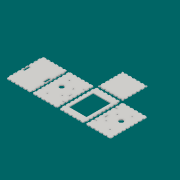
# Autodesk Inventor part: panelsWithKerf
Saved by Autodesk Inventor 2016 (Build 200138000, 138)
## iProperties
Created: 2016-09-07
Part Number: panelsWithKerf
Material: Generic
Document SubType Name: Modeling
Designer: sawaiz
Density: 1 g/cm^3
Appearance: Default
Author: sawaiz
Autodesk Inventor part; units mm, degrees
(part 1 of 2)
ref_plane "YZ Plane" through (0, 0, 0) normal (1, 0, 0) x (0, 1, 0)
ref_plane "XZ Plane" through (0, 0, 0) normal (0, 1, 0) x (-1, 0, 0)
ref_plane "XY Plane" through (0, 0, 0) normal (0, 0, 1) x (1, 0, 0)
sketch "Sketch2" plane through (0, 0, 0) normal (0, 0, 1) x (1, 0, 0)
  line L0 (-304.6687, 15) -> (-304.6687, -15) construction
  line L1 (-304.6687, -15) -> (-314.6687, -15) construction
  line L2 (-314.6687, -15) -> (-314.6687, 15) construction
  line L3 (-314.6687, 15) -> (-304.6687, 15) construction
  line L4 (-204.6687, 15) -> (-204.6687, -15) construction
  line L5 (-204.6687, -15) -> (-214.6687, -15) construction
  line L6 (-214.6687, -15) -> (-214.6687, 15) construction
  line L7 (-214.6687, 15) -> (-204.6687, 15) construction
  circle A0 centre (-316.4937, -50) radius 1.7 projected
  circle A1 centre (-316.4937, 50) radius 1.7 projected
  circle A2 centre (-202.8437, -50) radius 1.7 projected
  circle A3 centre (-202.8437, 50) radius 1.7 projected
  line L8 (-316.4937, 86.825) -> (-316.4937, 75) construction
  line L9 (-316.4937, 75) -> (-319.6687, 75) construction
  line L10 (-319.6687, 75) -> (-319.6687, 65) construction
  line L11 (-319.6687, 65) -> (-316.4937, 65) construction
  line L12 (-316.4937, 65) -> (-316.4937, 55) construction
  line L13 (-316.4937, 55) -> (-319.6687, 55) construction
  line L14 (-319.6687, 55) -> (-319.6687, 45) construction
  line L15 (-319.6687, 45) -> (-316.4937, 45) construction
  line L16 (-316.4937, 45) -> (-316.4937, 35) construction
  line L17 (-316.4937, 35) -> (-319.6687, 35) construction
  line L18 (-319.6687, 35) -> (-319.6687, 25) construction
  line L19 (-319.6687, 25) -> (-316.4937, 25) construction
  line L20 (-316.4937, 25) -> (-316.4937, 15) construction
  line L21 (-316.4937, 15) -> (-319.6687, 15) construction
  line L22 (-319.6687, 15) -> (-319.6687, 5) construction
  line L23 (-319.6687, 5) -> (-316.4937, 5) construction
  line L24 (-316.4937, 5) -> (-316.4937, -5) construction
  line L25 (-316.4937, -5) -> (-319.6687, -5) construction
  line L26 (-319.6687, -5) -> (-319.6687, -15) construction
  line L27 (-319.6687, -15) -> (-316.4937, -15) construction
  line L28 (-316.4937, -15) -> (-316.4937, -25) construction
  line L29 (-316.4937, -25) -> (-319.6687, -25) construction
  line L30 (-319.6687, -25) -> (-319.6687, -35) construction
  line L31 (-319.6687, -35) -> (-316.4937, -35) construction
  line L32 (-316.4937, -35) -> (-316.4937, -45) construction
  line L33 (-316.4937, -45) -> (-319.6687, -45) construction
  line L34 (-319.6687, -45) -> (-319.6687, -55) construction
  line L35 (-319.6687, -55) -> (-316.4937, -55) construction
  line L36 (-316.4937, -55) -> (-316.4937, -65) construction
  line L37 (-316.4937, -65) -> (-319.6687, -65) construction
  line L38 (-319.6687, -65) -> (-319.6687, -75) construction
  line L39 (-319.6687, -75) -> (-316.4937, -75) construction
  line L40 (-316.4937, -75) -> (-316.4937, -86.825) construction
  line L41 (-316.4937, -86.825) -> (-314.6687, -86.825) construction
  line L42 (-314.6687, -86.825) -> (-314.6687, -90) construction
  line L43 (-314.6687, -90) -> (-304.6687, -90) construction
  line L44 (-304.6687, -90) -> (-304.6687, -86.825) construction
  line L45 (-304.6687, -86.825) -> (-294.6687, -86.825) construction
  line L46 (-294.6687, -86.825) -> (-294.6687, -90) construction
  line L47 (-294.6687, -90) -> (-284.6687, -90) construction
  line L48 (-284.6687, -90) -> (-284.6687, -86.825) construction
  line L49 (-284.6687, -86.825) -> (-274.6687, -86.825) construction
  line L50 (-274.6687, -86.825) -> (-274.6687, -90) construction
  line L51 (-274.6687, -90) -> (-264.6687, -90) construction
  line L52 (-264.6687, -90) -> (-264.6687, -86.825) construction
  line L53 (-264.6687, -86.825) -> (-254.6687, -86.825) construction
  line L54 (-254.6687, -86.825) -> (-254.6687, -90) construction
  line L55 (-254.6687, -90) -> (-244.6687, -90) construction
  line L56 (-244.6687, -90) -> (-244.6687, -86.825) construction
  line L57 (-244.6687, -86.825) -> (-234.6687, -86.825) construction
  line L58 (-234.6687, -86.825) -> (-234.6687, -90) construction
  line L59 (-234.6687, -90) -> (-224.6687, -90) construction
  line L60 (-224.6687, -90) -> (-224.6687, -86.825) construction
  line L61 (-224.6687, -86.825) -> (-214.6687, -86.825) construction
  line L62 (-214.6687, -86.825) -> (-214.6687, -90) construction
  line L63 (-214.6687, -90) -> (-204.6687, -90) construction
  line L64 (-204.6687, -90) -> (-204.6687, -86.825) construction
  line L65 (-204.6687, -86.825) -> (-202.8437, -86.825) construction
  line L66 (-202.8437, -86.825) -> (-202.8437, -75) construction
  line L67 (-202.8437, -75) -> (-199.6687, -75) construction
  line L68 (-199.6687, -75) -> (-199.6687, -65) construction
  line L69 (-199.6687, -65) -> (-202.8437, -65) construction
  line L70 (-202.8437, -65) -> (-202.8437, -55) construction
  line L71 (-202.8437, -55) -> (-199.6687, -55) construction
  line L72 (-199.6687, -55) -> (-199.6687, -45) construction
  line L73 (-199.6687, -45) -> (-202.8437, -45) construction
  line L74 (-202.8437, -45) -> (-202.8437, -35) construction
  line L75 (-202.8437, -35) -> (-199.6687, -35) construction
  line L76 (-199.6687, -35) -> (-199.6687, -25) construction
  line L77 (-199.6687, -25) -> (-202.8437, -25) construction
  line L78 (-202.8437, -25) -> (-202.8437, -15) construction
  line L79 (-202.8437, -15) -> (-199.6687, -15) construction
  line L80 (-199.6687, -15) -> (-199.6687, -5) construction
  line L81 (-199.6687, -5) -> (-202.8437, -5) construction
  line L82 (-202.8437, -5) -> (-202.8437, 5) construction
  line L83 (-202.8437, 5) -> (-199.6687, 5) construction
  line L84 (-199.6687, 5) -> (-199.6687, 15) construction
  line L85 (-199.6687, 15) -> (-202.8437, 15) construction
  line L86 (-202.8437, 15) -> (-202.8437, 25) construction
  line L87 (-202.8437, 25) -> (-199.6687, 25) construction
  line L88 (-199.6687, 25) -> (-199.6687, 35) construction
  line L89 (-199.6687, 35) -> (-202.8437, 35) construction
  line L90 (-202.8437, 35) -> (-202.8437, 45) construction
  line L91 (-202.8437, 45) -> (-199.6687, 45) construction
  line L92 (-199.6687, 45) -> (-199.6687, 55) construction
  line L93 (-199.6687, 55) -> (-202.8437, 55) construction
  line L94 (-202.8437, 55) -> (-202.8437, 65) construction
  line L95 (-202.8437, 65) -> (-199.6687, 65) construction
  line L96 (-199.6687, 65) -> (-199.6687, 75) construction
  line L97 (-199.6687, 75) -> (-202.8437, 75) construction
  line L98 (-202.8437, 75) -> (-202.8437, 86.825) construction
  line L99 (-202.8437, 86.825) -> (-204.6687, 86.825) construction
  line L100 (-204.6687, 86.825) -> (-204.6687, 90) construction
  line L101 (-204.6687, 90) -> (-214.6687, 90) construction
  line L102 (-214.6687, 90) -> (-214.6687, 86.825) construction
  line L103 (-214.6687, 86.825) -> (-224.6687, 86.825) construction
  line L104 (-224.6687, 86.825) -> (-224.6687, 90) construction
  line L105 (-224.6687, 90) -> (-234.6687, 90) construction
  line L106 (-234.6687, 90) -> (-234.6687, 86.825) construction
  line L107 (-234.6687, 86.825) -> (-244.6687, 86.825) construction
  line L108 (-244.6687, 86.825) -> (-244.6687, 90) construction
  line L109 (-244.6687, 90) -> (-254.6687, 90) construction
  line L110 (-254.6687, 90) -> (-254.6687, 86.825) construction
  line L111 (-254.6687, 86.825) -> (-264.6687, 86.825) construction
  line L112 (-264.6687, 86.825) -> (-264.6687, 90) construction
  line L113 (-264.6687, 90) -> (-274.6687, 90) construction
  line L114 (-274.6687, 90) -> (-274.6687, 86.825) construction
  line L115 (-274.6687, 86.825) -> (-284.6687, 86.825) construction
  line L116 (-284.6687, 86.825) -> (-284.6687, 90) construction
  line L117 (-284.6687, 90) -> (-294.6687, 90) construction
  line L118 (-294.6687, 90) -> (-294.6687, 86.825) construction
  line L119 (-294.6687, 86.825) -> (-304.6687, 86.825) construction
  line L120 (-304.6687, 86.825) -> (-304.6687, 90) construction
  line L121 (-304.6687, 90) -> (-314.6687, 90) construction
  line L122 (-314.6687, 90) -> (-314.6687, 86.825) construction
  line L123 (-314.6687, 86.825) -> (-316.4937, 86.825) construction
  line L124 (-87.1256, -13.335) -> (-90.9356, -13.335) projected
  line L125 (-90.9356, -13.335) -> (-90.9356, -1.905) projected
  line L126 (-90.9356, -1.905) -> (-87.1256, -1.905) projected
  line L127 (-87.1256, -1.905) -> (-87.1256, -13.335) projected
  circle A4 centre (-92.8406, -15.24) radius 1.078 projected
  circle A5 centre (-85.2206, 0) radius 1.078 projected
  circle A6 centre (-85.2206, -15.24) radius 1.078 projected
  circle A7 centre (-92.8406, 0) radius 1.078 projected
  line L128 (-76.1156, -48.5) -> (-74.1156, -48.5) construction
  line L129 (-74.1156, -48.5) -> (-74.1156, -45) construction
  line L130 (-74.1156, -45) -> (-70.9406, -45) construction
  line L131 (-70.9406, -45) -> (-70.9406, -35) construction
  line L132 (-70.9406, -35) -> (-74.1156, -35) construction
  line L133 (-74.1156, -35) -> (-74.1156, -25) construction
  line L134 (-74.1156, -25) -> (-70.9406, -25) construction
  line L135 (-70.9406, -25) -> (-70.9406, -15) construction
  line L136 (-70.9406, -15) -> (-74.1156, -15) construction
  line L137 (-74.1156, -15) -> (-74.1156, -5) construction
  line L138 (-74.1156, -5) -> (-70.9406, -5) construction
  line L139 (-70.9406, -5) -> (-70.9406, 5) construction
  line L140 (-70.9406, 5) -> (-74.1156, 5) construction
  line L141 (-74.1156, 5) -> (-74.1156, 15) construction
  line L142 (-74.1156, 15) -> (-70.9406, 15) construction
  line L143 (-70.9406, 15) -> (-70.9406, 25) construction
  line L144 (-70.9406, 25) -> (-74.1156, 25) construction
  line L145 (-74.1156, 25) -> (-74.1156, 35) construction
  line L146 (-74.1156, 35) -> (-70.9406, 35) construction
  line L147 (-70.9406, 35) -> (-70.9406, 45) construction
  line L148 (-70.9406, 45) -> (-74.1156, 45) construction
  line L149 (-74.1156, 45) -> (-74.1156, 48.5) construction
  line L150 (-74.1156, 48.5) -> (-76.1156, 48.5) construction
  line L151 (-76.1156, 48.5) -> (-76.1156, 47.25) construction
  line L152 (-76.1156, 47.25) -> (-78.6156, 47.25) construction
  line L153 (-78.6156, 47.25) -> (-78.6156, 48.5) construction
  line L154 (-78.6156, 48.5) -> (-84.9406, 48.5) construction
  line L155 (-84.9406, 48.5) -> (-84.9406, 51.5) construction
  line L156 (-84.9406, 51.5) -> (-78.6156, 51.5) construction
  line L157 (-78.6156, 51.5) -> (-78.6156, 52.75) construction
  line L158 (-78.6156, 52.75) -> (-76.1156, 52.75) construction
  line L159 (-76.1156, 52.75) -> (-76.1156, 51.5) construction
  line L160 (-76.1156, 51.5) -> (-74.1156, 51.5) construction
  line L161 (-74.1156, 51.5) -> (-74.1156, 55) construction
  line L162 (-74.1156, 55) -> (-70.9406, 55) construction
  line L163 (-70.9406, 55) -> (-70.9406, 65) construction
  line L164 (-70.9406, 65) -> (-74.1156, 65) construction
  line L165 (-74.1156, 65) -> (-74.1156, 75) construction
  line L166 (-74.1156, 75) -> (-70.9406, 75) construction
  line L167 (-70.9406, 75) -> (-70.9406, 86.825) construction
  line L168 (-75.9406, 86.825) -> (-70.9406, 86.825) construction
  line L169 (-75.9406, 90) -> (-75.9406, 86.825) construction
  line L170 (-85.9406, 90) -> (-75.9406, 90) construction
  line L171 (-85.9406, 86.825) -> (-85.9406, 90) construction
  line L172 (-85.9406, 86.825) -> (-95.9406, 86.825) construction
  line L173 (-95.9406, 90) -> (-95.9406, 86.825) construction
  line L174 (-105.9406, 90) -> (-95.9406, 90) construction
  line L175 (-105.9406, 86.825) -> (-105.9406, 90) construction
  line L176 (-105.9406, 86.825) -> (-115.9406, 86.825) construction
  line L177 (-115.9406, 90) -> (-115.9406, 86.825) construction
  line L178 (-125.9406, 90) -> (-115.9406, 90) construction
  line L179 (-125.9406, 86.825) -> (-125.9406, 90) construction
  line L180 (-125.9406, 86.825) -> (-135.9406, 86.825) construction
  line L181 (-135.9406, 90) -> (-135.9406, 86.825) construction
  line L182 (-145.9406, 90) -> (-135.9406, 90) construction
  line L183 (-145.9406, 86.825) -> (-145.9406, 90) construction
  line L184 (-145.9406, 86.825) -> (-155.9406, 86.825) construction
  line L185 (-155.9406, 90) -> (-155.9406, 86.825) construction
  line L186 (-165.9406, 90) -> (-155.9406, 90) construction
  line L187 (-165.9406, 86.825) -> (-165.9406, 90) construction
  line L188 (-165.9406, 86.825) -> (-175.9406, 86.825) construction
  line L189 (-175.9406, 90) -> (-175.9406, 86.825) construction
  line L190 (-185.9406, 90) -> (-175.9406, 90) construction
  line L191 (-185.9406, 86.825) -> (-185.9406, 90) construction
  line L192 (-185.9406, 86.825) -> (-190.9406, 86.825) construction
  line L193 (-190.9406, 75) -> (-190.9406, 86.825) construction
  line L194 (-187.7656, 75) -> (-190.9406, 75) construction
  line L195 (-187.7656, 75) -> (-187.7656, 65) construction
  line L196 (-190.9406, 65) -> (-187.7656, 65) construction
  line L197 (-190.9406, 55) -> (-190.9406, 65) construction
  line L198 (-187.7656, 55) -> (-190.9406, 55) construction
  line L199 (-187.7656, 55) -> (-187.7656, 45) construction
  line L200 (-190.9406, 45) -> (-187.7656, 45) construction
  line L201 (-190.9406, 35) -> (-190.9406, 45) construction
  line L202 (-187.7656, 35) -> (-190.9406, 35) construction
  line L203 (-187.7656, 35) -> (-187.7656, 25) construction
  line L204 (-190.9406, 25) -> (-187.7656, 25) construction
  line L205 (-190.9406, 15) -> (-190.9406, 25) construction
  line L206 (-187.7656, 15) -> (-190.9406, 15) construction
  line L207 (-187.7656, 15) -> (-187.7656, 5) construction
  line L208 (-190.9406, 5) -> (-187.7656, 5) construction
  line L209 (-190.9406, -5) -> (-190.9406, 5) construction
  line L210 (-187.7656, -5) -> (-190.9406, -5) construction
  line L211 (-187.7656, -5) -> (-187.7656, -15) construction
  line L212 (-190.9406, -15) -> (-187.7656, -15) construction
  line L213 (-190.9406, -25) -> (-190.9406, -15) construction
  line L214 (-187.7656, -25) -> (-190.9406, -25) construction
  line L215 (-187.7656, -25) -> (-187.7656, -35) construction
  line L216 (-190.9406, -35) -> (-187.7656, -35) construction
  line L217 (-190.9406, -45) -> (-190.9406, -35) construction
  line L218 (-187.7656, -45) -> (-190.9406, -45) construction
  line L219 (-187.7656, -45) -> (-187.7656, -55) construction
  line L220 (-190.9406, -55) -> (-187.7656, -55) construction
  line L221 (-190.9406, -65) -> (-190.9406, -55) construction
  line L222 (-187.7656, -65) -> (-190.9406, -65) construction
  line L223 (-187.7656, -65) -> (-187.7656, -75) construction
  line L224 (-190.9406, -75) -> (-187.7656, -75) construction
  line L225 (-190.9406, -75) -> (-190.9406, -86.825) construction
  line L226 (-190.9406, -86.825) -> (-185.9406, -86.825) construction
  line L227 (-185.9406, -86.825) -> (-185.9406, -90) construction
  line L228 (-185.9406, -90) -> (-175.9406, -90) construction
  line L229 (-175.9406, -90) -> (-175.9406, -86.825) construction
  line L230 (-175.9406, -86.825) -> (-165.9406, -86.825) construction
  line L231 (-165.9406, -86.825) -> (-165.9406, -90) construction
  line L232 (-165.9406, -90) -> (-155.9406, -90) construction
  line L233 (-155.9406, -90) -> (-155.9406, -86.825) construction
  line L234 (-155.9406, -86.825) -> (-145.9406, -86.825) construction
  line L235 (-145.9406, -86.825) -> (-145.9406, -90) construction
  line L236 (-145.9406, -90) -> (-135.9406, -90) construction
  line L237 (-135.9406, -90) -> (-135.9406, -86.825) construction
  line L238 (-135.9406, -86.825) -> (-125.9406, -86.825) construction
  line L239 (-125.9406, -86.825) -> (-125.9406, -90) construction
  line L240 (-125.9406, -90) -> (-115.9406, -90) construction
  line L241 (-115.9406, -90) -> (-115.9406, -86.825) construction
  line L242 (-115.9406, -86.825) -> (-105.9406, -86.825) construction
  line L243 (-105.9406, -86.825) -> (-105.9406, -90) construction
  line L244 (-105.9406, -90) -> (-95.9406, -90) construction
  line L245 (-95.9406, -90) -> (-95.9406, -86.825) construction
  line L246 (-95.9406, -86.825) -> (-85.9406, -86.825) construction
  line L247 (-85.9406, -86.825) -> (-85.9406, -90) construction
  line L248 (-85.9406, -90) -> (-75.9406, -90) construction
  line L249 (-75.9406, -90) -> (-75.9406, -86.825) construction
  line L250 (-75.9406, -86.825) -> (-70.9406, -86.825) construction
  line L251 (-70.9406, -86.825) -> (-70.9406, -75) construction
  line L252 (-70.9406, -75) -> (-74.1156, -75) construction
  line L253 (-74.1156, -75) -> (-74.1156, -65) construction
  line L254 (-74.1156, -65) -> (-70.9406, -65) construction
  line L255 (-70.9406, -65) -> (-70.9406, -55) construction
  line L256 (-70.9406, -55) -> (-74.1156, -55) construction
  line L257 (-74.1156, -55) -> (-74.1156, -51.5) construction
  line L258 (-74.1156, -51.5) -> (-76.1156, -51.5) construction
  line L259 (-76.1156, -51.5) -> (-76.1156, -52.75) construction
  line L260 (-76.1156, -52.75) -> (-78.6156, -52.75) construction
  line L261 (-78.6156, -52.75) -> (-78.6156, -51.5) construction
  line L262 (-78.6156, -51.5) -> (-84.9406, -51.5) construction
  line L263 (-84.9406, -51.5) -> (-84.9406, -48.5) construction
  line L264 (-84.9406, -48.5) -> (-78.6156, -48.5) construction
  line L265 (-78.6156, -48.5) -> (-78.6156, -47.25) construction
  line L266 (-78.6156, -47.25) -> (-76.1156, -47.25) construction
  line L267 (-76.1156, -47.25) -> (-76.1156, -48.5) construction
  circle A8 centre (-107.9434, -27.4451) radius 3 projected
  circle A9 centre (-153.9378, 54) radius 3 projected
  circle A10 centre (-107.9434, 27.4451) radius 3 projected
  circle A11 centre (-153.9378, -54) radius 3 projected
  circle A12 centre (-145.9406, 8.175) radius 11 projected
  line L268 (43.8, 60) -> (43.8, -60) construction
  line L269 (43.8, -60) -> (-43.8, -60) construction
  line L270 (-43.8, -60) -> (-43.8, 60) construction
  line L271 (-43.8, 60) -> (43.8, 60) construction
  line L272 (-56.825, 86.825) -> (-56.825, 75) construction
  line L273 (-56.825, 75) -> (-60, 75) construction
  line L274 (-60, 75) -> (-60, 65) construction
  line L275 (-60, 65) -> (-56.825, 65) construction
  line L276 (-56.825, 65) -> (-56.825, 55) construction
  line L277 (-56.825, 55) -> (-60, 55) construction
  line L278 (-60, 55) -> (-60, 45) construction
  line L279 (-60, 45) -> (-56.825, 45) construction
  line L280 (-56.825, 45) -> (-56.825, 35) construction
  line L281 (-56.825, 35) -> (-60, 35) construction
  line L282 (-60, 35) -> (-60, 25) construction
  line L283 (-60, 25) -> (-56.825, 25) construction
  line L284 (-56.825, 25) -> (-56.825, 15) construction
  line L285 (-56.825, 15) -> (-60, 15) construction
  line L286 (-60, 15) -> (-60, 5) construction
  line L287 (-60, 5) -> (-56.825, 5) construction
  line L288 (-56.825, 5) -> (-56.825, -5) construction
  line L289 (-56.825, -5) -> (-60, -5) construction
  line L290 (-60, -5) -> (-60, -15) construction
  line L291 (-60, -15) -> (-56.825, -15) construction
  line L292 (-56.825, -15) -> (-56.825, -25) construction
  line L293 (-56.825, -25) -> (-60, -25) construction
  line L294 (-60, -25) -> (-60, -35) construction
  line L295 (-60, -35) -> (-56.825, -35) construction
  line L296 (-56.825, -35) -> (-56.825, -45) construction
  line L297 (-56.825, -45) -> (-60, -45) construction
  line L298 (-60, -45) -> (-60, -55) construction
  line L299 (-60, -55) -> (-56.825, -55) construction
  line L300 (-56.825, -55) -> (-56.825, -65) construction
  line L301 (-56.825, -65) -> (-60, -65) construction
  line L302 (-60, -65) -> (-60, -75) construction
  line L303 (-60, -75) -> (-56.825, -75) construction
  line L304 (-56.825, -75) -> (-56.825, -86.825) construction
  line L305 (-56.825, -86.825) -> (-55, -86.825) construction
  line L306 (-55, -86.825) -> (-55, -90) construction
  line L307 (-55, -90) -> (-45, -90) construction
  line L308 (-45, -90) -> (-45, -86.825) construction
  line L309 (-45, -86.825) -> (-35, -86.825) construction
  line L310 (-35, -86.825) -> (-35, -90) construction
  line L311 (-35, -90) -> (-25, -90) construction
  line L312 (-25, -90) -> (-25, -86.825) construction
  line L313 (-25, -86.825) -> (-15, -86.825) construction
  line L314 (-15, -86.825) -> (-15, -90) construction
  line L315 (-15, -90) -> (-5, -90) construction
  line L316 (-5, -90) -> (-5, -86.825) construction
  line L317 (-5, -86.825) -> (5, -86.825) construction
  line L318 (5, -86.825) -> (5, -90) construction
  line L319 (5, -90) -> (15, -90) construction
  line L320 (15, -90) -> (15, -86.825) construction
  line L321 (15, -86.825) -> (25, -86.825) construction
  line L322 (25, -86.825) -> (25, -90) construction
  line L323 (25, -90) -> (35, -90) construction
  line L324 (35, -90) -> (35, -86.825) construction
  line L325 (35, -86.825) -> (45, -86.825) construction
  line L326 (45, -86.825) -> (45, -90) construction
  line L327 (45, -90) -> (55, -90) construction
  line L328 (55, -90) -> (55, -86.825) construction
  line L329 (55, -86.825) -> (56.825, -86.825) construction
  line L330 (56.825, -86.825) -> (56.825, -75) construction
  line L331 (56.825, -75) -> (60, -75) construction
  line L332 (60, -75) -> (60, -65) construction
  line L333 (60, -65) -> (56.825, -65) construction
  line L334 (56.825, -65) -> (56.825, -55) construction
  line L335 (56.825, -55) -> (60, -55) construction
  line L336 (60, -55) -> (60, -45) construction
  line L337 (60, -45) -> (56.825, -45) construction
  line L338 (56.825, -45) -> (56.825, -35) construction
  line L339 (56.825, -35) -> (60, -35) construction
  line L340 (60, -35) -> (60, -25) construction
  line L341 (60, -25) -> (56.825, -25) construction
  line L342 (56.825, -25) -> (56.825, -15) construction
  line L343 (56.825, -15) -> (60, -15) construction
  line L344 (60, -15) -> (60, -5) construction
  line L345 (60, -5) -> (56.825, -5) construction
  line L346 (56.825, -5) -> (56.825, 5) construction
  line L347 (56.825, 5) -> (60, 5) construction
  line L348 (60, 5) -> (60, 15) construction
  line L349 (60, 15) -> (56.825, 15) construction
  line L350 (56.825, 15) -> (56.825, 25) construction
  line L351 (56.825, 25) -> (60, 25) construction
  line L352 (60, 25) -> (60, 35) construction
  line L353 (60, 35) -> (56.825, 35) construction
  line L354 (56.825, 35) -> (56.825, 45) construction
  line L355 (56.825, 45) -> (60, 45) construction
  line L356 (60, 45) -> (60, 55) construction
  line L357 (60, 55) -> (56.825, 55) construction
  line L358 (56.825, 55) -> (56.825, 65) construction
  line L359 (56.825, 65) -> (60, 65) construction
  line L360 (60, 65) -> (60, 75) construction
  line L361 (60, 75) -> (56.825, 75) construction
  line L362 (56.825, 75) -> (56.825, 86.825) construction
  line L363 (56.825, 86.825) -> (55, 86.825) construction
  line L364 (55, 86.825) -> (55, 90) construction
  line L365 (55, 90) -> (45, 90) construction
  line L366 (45, 90) -> (45, 86.825) construction
  line L367 (45, 86.825) -> (35, 86.825) construction
  line L368 (35, 86.825) -> (35, 90) construction
  line L369 (35, 90) -> (25, 90) construction
  line L370 (25, 90) -> (25, 86.825) construction
  line L371 (25, 86.825) -> (15, 86.825) construction
  line L372 (15, 86.825) -> (15, 90) construction
  line L373 (15, 90) -> (5, 90) construction
  line L374 (5, 90) -> (5, 86.825) construction
  line L375 (5, 86.825) -> (-5, 86.825) construction
  line L376 (-5, 86.825) -> (-5, 90) construction
  line L377 (-5, 90) -> (-15, 90) construction
  line L378 (-15, 90) -> (-15, 86.825) construction
  line L379 (-15, 86.825) -> (-25, 86.825) construction
  line L380 (-25, 86.825) -> (-25, 90) construction
  line L381 (-25, 90) -> (-35, 90) construction
  line L382 (-35, 90) -> (-35, 86.825) construction
  line L383 (-35, 86.825) -> (-45, 86.825) construction
  line L384 (-45, 86.825) -> (-45, 90) construction
  line L385 (-45, 90) -> (-55, 90) construction
  line L386 (-55, 90) -> (-55, 86.825) construction
  line L387 (-55, 86.825) -> (-56.825, 86.825) construction
  line L388 (56.825, 215.8646) -> (60, 215.8646) construction
  line L389 (60, 215.8646) -> (60, 220.8646) construction
  line L390 (60, 220.8646) -> (55, 220.8646) construction
  line L391 (55, 220.8646) -> (55, 217.6896) construction
  line L392 (55, 217.6896) -> (45, 217.6896) construction
  line L393 (45, 217.6896) -> (45, 220.8646) construction
  line L394 (45, 220.8646) -> (35, 220.8646) construction
  line L395 (35, 220.8646) -> (35, 217.6896) construction
  line L396 (35, 217.6896) -> (25, 217.6896) construction
  line L397 (25, 217.6896) -> (25, 220.8646) construction
  line L398 (25, 220.8646) -> (15, 220.8646) construction
  line L399 (15, 220.8646) -> (15, 217.6896) construction
  line L400 (15, 217.6896) -> (5, 217.6896) construction
  line L401 (5, 217.6896) -> (5, 220.8646) construction
  line L402 (5, 220.8646) -> (-5, 220.8646) construction
  line L403 (-5, 220.8646) -> (-5, 217.6896) construction
  line L404 (-5, 217.6896) -> (-15, 217.6896) construction
  line L405 (-15, 217.6896) -> (-15, 220.8646) construction
  line L406 (-15, 220.8646) -> (-25, 220.8646) construction
  line L407 (-25, 220.8646) -> (-25, 217.6896) construction
  line L408 (-25, 217.6896) -> (-35, 217.6896) construction
  line L409 (-35, 217.6896) -> (-35, 220.8646) construction
  line L410 (-35, 220.8646) -> (-45, 220.8646) construction
  line L411 (-45, 220.8646) -> (-45, 217.6896) construction
  line L412 (-45, 217.6896) -> (-55, 217.6896) construction
  line L413 (-55, 217.6896) -> (-55, 220.8646) construction
  line L414 (-55, 220.8646) -> (-60, 220.8646) construction
  line L415 (-60, 220.8646) -> (-60, 215.8646) construction
  line L416 (-60, 215.8646) -> (-56.825, 215.8646) construction
  line L417 (-56.825, 215.8646) -> (-56.825, 205.8646) construction
  line L418 (-56.825, 205.8646) -> (-60, 205.8646) construction
  line L419 (-60, 205.8646) -> (-60, 195.8646) construction
  line L420 (-60, 195.8646) -> (-56.825, 195.8646) construction
  line L421 (-56.825, 195.8646) -> (-56.825, 185.8646) construction
  line L422 (-56.825, 185.8646) -> (-60, 185.8646) construction
  line L423 (-60, 185.8646) -> (-60, 175.8646) construction
  line L424 (-60, 175.8646) -> (-56.825, 175.8646) construction
  line L425 (-56.825, 175.8646) -> (-56.825, 165.8646) construction
  line L426 (-56.825, 165.8646) -> (-60, 165.8646) construction
  line L427 (-60, 165.8646) -> (-60, 155.8646) construction
  line L428 (-60, 155.8646) -> (-56.825, 155.8646) construction
  line L429 (-56.825, 155.8646) -> (-56.825, 145.8646) construction
  line L430 (-56.825, 145.8646) -> (-60, 145.8646) construction
  line L431 (-60, 145.8646) -> (-60, 135.8646) construction
  line L432 (-60, 135.8646) -> (-56.825, 135.8646) construction
  line L433 (-56.825, 135.8646) -> (-56.825, 125.8646) construction
  line L434 (-56.825, 125.8646) -> (-60, 125.8646) construction
  line L435 (-60, 125.8646) -> (-60, 115.8646) construction
  line L436 (-60, 115.8646) -> (-56.825, 115.8646) construction
  line L437 (-56.825, 115.8646) -> (-56.825, 105.8646) construction
  line L438 (-56.825, 105.8646) -> (-60, 105.8646) construction
  line L439 (-60, 105.8646) -> (-60, 100.8646) construction
  line L440 (-60, 100.8646) -> (-55, 100.8646) construction
  line L441 (-55, 100.8646) -> (-55, 104.0396) construction
  line L442 (-55, 104.0396) -> (-45, 104.0396) construction
  line L443 (-45, 104.0396) -> (-45, 100.8646) construction
  line L444 (-45, 100.8646) -> (-35, 100.8646) construction
  line L445 (-35, 100.8646) -> (-35, 104.0396) construction
  line L446 (-35, 104.0396) -> (-25, 104.0396) construction
  line L447 (-25, 104.0396) -> (-25, 100.8646) construction
  line L448 (-25, 100.8646) -> (-15, 100.8646) construction
  line L449 (-15, 100.8646) -> (-15, 104.0396) construction
  line L450 (-15, 104.0396) -> (-5, 104.0396) construction
  line L451 (-5, 104.0396) -> (-5, 100.8646) construction
  line L452 (-5, 100.8646) -> (5, 100.8646) construction
  line L453 (5, 100.8646) -> (5, 104.0396) construction
  line L454 (5, 104.0396) -> (15, 104.0396) construction
  line L455 (15, 104.0396) -> (15, 100.8646) construction
  line L456 (15, 100.8646) -> (25, 100.8646) construction
  line L457 (25, 100.8646) -> (25, 104.0396) construction
  line L458 (25, 104.0396) -> (35, 104.0396) construction
  line L459 (35, 104.0396) -> (35, 100.8646) construction
  line L460 (35, 100.8646) -> (45, 100.8646) construction
  line L461 (45, 100.8646) -> (45, 104.0396) construction
  line L462 (45, 104.0396) -> (55, 104.0396) construction
  line L463 (55, 104.0396) -> (55, 100.8646) construction
  line L464 (55, 100.8646) -> (60, 100.8646) construction
  line L465 (60, 100.8646) -> (60, 105.8646) construction
  line L466 (60, 105.8646) -> (56.825, 105.8646) construction
  line L467 (56.825, 105.8646) -> (56.825, 115.8646) construction
  line L468 (56.825, 115.8646) -> (60, 115.8646) construction
  line L469 (60, 115.8646) -> (60, 125.8646) construction
  line L470 (60, 125.8646) -> (56.825, 125.8646) construction
  line L471 (56.825, 125.8646) -> (56.825, 135.8646) construction
  line L472 (56.825, 135.8646) -> (60, 135.8646) construction
  line L473 (60, 135.8646) -> (60, 145.8646) construction
  line L474 (60, 145.8646) -> (56.825, 145.8646) construction
  line L475 (56.825, 145.8646) -> (56.825, 155.8646) construction
  line L476 (56.825, 155.8646) -> (60, 155.8646) construction
  line L477 (60, 155.8646) -> (60, 165.8646) construction
  line L478 (60, 165.8646) -> (56.825, 165.8646) construction
  line L479 (56.825, 165.8646) -> (56.825, 175.8646) construction
  line L480 (56.825, 175.8646) -> (60, 175.8646) construction
  line L481 (60, 175.8646) -> (60, 185.8646) construction
  line L482 (60, 185.8646) -> (56.825, 185.8646) construction
  line L483 (56.825, 185.8646) -> (56.825, 195.8646) construction
  line L484 (56.825, 195.8646) -> (60, 195.8646) construction
  line L485 (60, 195.8646) -> (60, 205.8646) construction
  line L486 (60, 205.8646) -> (56.825, 205.8646) construction
  line L487 (56.825, 205.8646) -> (56.825, 215.8646) construction
  line L488 (90.1923, -13.335) -> (86.3823, -13.335) projected
  line L489 (86.3823, -13.335) -> (86.3823, -1.905) projected
  line L490 (86.3823, -1.905) -> (90.1923, -1.905) projected
  line L491 (90.1923, -1.905) -> (90.1923, -13.335) projected
  circle A13 centre (92.0973, -15.24) radius 1.078 projected
  circle A14 centre (84.4773, 0) radius 1.078 projected
  circle A15 centre (84.4773, -15.24) radius 1.078 projected
  circle A16 centre (92.0973, 0) radius 1.078 projected
  circle A17 centre (107.2001, -27.4451) radius 3 projected
  circle A18 centre (153.1945, 54) radius 3 projected
  circle A19 centre (107.2001, 27.4451) radius 3 projected
  circle A20 centre (153.1945, -54) radius 3 projected
  circle A21 centre (145.1973, 8.175) radius 11 projected
  line L492 (73.3723, -48.5) -> (75.3723, -48.5) construction
  line L493 (75.3723, -48.5) -> (75.3723, -47.25) construction
  line L494 (75.3723, -47.25) -> (77.8723, -47.25) construction
  line L495 (77.8723, -47.25) -> (77.8723, -48.5) construction
  line L496 (77.8723, -48.5) -> (84.1973, -48.5) construction
  line L497 (84.1973, -48.5) -> (84.1973, -51.5) construction
  line L498 (84.1973, -51.5) -> (77.8723, -51.5) construction
  line L499 (77.8723, -51.5) -> (77.8723, -52.75) construction
  line L500 (77.8723, -52.75) -> (75.3723, -52.75) construction
  line L501 (75.3723, -52.75) -> (75.3723, -51.5) construction
  line L502 (75.3723, -51.5) -> (73.3723, -51.5) construction
  line L503 (73.3723, -55) -> (73.3723, -51.5) construction
  line L504 (70.1973, -55) -> (73.3723, -55) construction
  line L505 (70.1973, -65) -> (70.1973, -55) construction
  line L506 (73.3723, -65) -> (70.1973, -65) construction
  line L507 (73.3723, -75) -> (73.3723, -65) construction
  line L508 (70.1973, -75) -> (73.3723, -75) construction
  line L509 (70.1973, -86.825) -> (70.1973, -75) construction
  line L510 (75.1973, -86.825) -> (70.1973, -86.825) construction
  line L511 (75.1973, -90) -> (75.1973, -86.825) construction
  line L512 (85.1973, -90) -> (75.1973, -90) construction
  line L513 (85.1973, -86.825) -> (85.1973, -90) construction
  line L514 (95.1973, -86.825) -> (85.1973, -86.825) construction
  line L515 (95.1973, -90) -> (95.1973, -86.825) construction
  line L516 (105.1973, -90) -> (95.1973, -90) construction
  line L517 (105.1973, -86.825) -> (105.1973, -90) construction
  line L518 (115.1973, -86.825) -> (105.1973, -86.825) construction
  line L519 (115.1973, -90) -> (115.1973, -86.825) construction
  line L520 (125.1973, -90) -> (115.1973, -90) construction
  line L521 (125.1973, -86.825) -> (125.1973, -90) construction
  line L522 (135.1973, -86.825) -> (125.1973, -86.825) construction
  line L523 (135.1973, -90) -> (135.1973, -86.825) construction
  line L524 (145.1973, -90) -> (135.1973, -90) construction
  line L525 (145.1973, -86.825) -> (145.1973, -90) construction
  line L526 (155.1973, -86.825) -> (145.1973, -86.825) construction
  line L527 (155.1973, -90) -> (155.1973, -86.825) construction
  line L528 (165.1973, -90) -> (155.1973, -90) construction
  line L529 (165.1973, -86.825) -> (165.1973, -90) construction
  line L530 (175.1973, -86.825) -> (165.1973, -86.825) construction
  line L531 (175.1973, -90) -> (175.1973, -86.825) construction
  line L532 (185.1973, -90) -> (175.1973, -90) construction
  line L533 (185.1973, -86.825) -> (185.1973, -90) construction
  line L534 (190.1973, -86.825) -> (185.1973, -86.825) construction
  line L535 (190.1973, -86.825) -> (190.1973, -75) construction
  line L536 (190.1973, -75) -> (187.0223, -75) construction
  line L537 (187.0223, -65) -> (187.0223, -75) construction
  line L538 (187.0223, -65) -> (190.1973, -65) construction
  line L539 (190.1973, -65) -> (190.1973, -55) construction
  line L540 (190.1973, -55) -> (187.0223, -55) construction
  line L541 (187.0223, -45) -> (187.0223, -55) construction
  line L542 (187.0223, -45) -> (190.1973, -45) construction
  line L543 (190.1973, -45) -> (190.1973, -35) construction
  line L544 (190.1973, -35) -> (187.0223, -35) construction
  line L545 (187.0223, -25) -> (187.0223, -35) construction
  line L546 (187.0223, -25) -> (190.1973, -25) construction
  line L547 (190.1973, -25) -> (190.1973, -15) construction
  line L548 (190.1973, -15) -> (187.0223, -15) construction
  line L549 (187.0223, -5) -> (187.0223, -15) construction
  line L550 (187.0223, -5) -> (190.1973, -5) construction
  line L551 (190.1973, -5) -> (190.1973, 5) construction
  line L552 (190.1973, 5) -> (187.0223, 5) construction
  line L553 (187.0223, 15) -> (187.0223, 5) construction
  line L554 (187.0223, 15) -> (190.1973, 15) construction
  line L555 (190.1973, 15) -> (190.1973, 25) construction
  line L556 (190.1973, 25) -> (187.0223, 25) construction
  line L557 (187.0223, 35) -> (187.0223, 25) construction
  line L558 (187.0223, 35) -> (190.1973, 35) construction
  line L559 (190.1973, 35) -> (190.1973, 45) construction
  line L560 (190.1973, 45) -> (187.0223, 45) construction
  line L561 (187.0223, 55) -> (187.0223, 45) construction
  line L562 (187.0223, 55) -> (190.1973, 55) construction
  line L563 (190.1973, 55) -> (190.1973, 65) construction
  line L564 (190.1973, 65) -> (187.0223, 65) construction
  line L565 (187.0223, 75) -> (187.0223, 65) construction
  line L566 (187.0223, 75) -> (190.1973, 75) construction
  line L567 (190.1973, 75) -> (190.1973, 86.825) construction
  line L568 (185.1973, 86.825) -> (190.1973, 86.825) construction
  line L569 (185.1973, 86.825) -> (185.1973, 90) construction
  line L570 (185.1973, 90) -> (175.1973, 90) construction
  line L571 (175.1973, 90) -> (175.1973, 86.825) construction
  line L572 (165.1973, 86.825) -> (175.1973, 86.825) construction
  line L573 (165.1973, 86.825) -> (165.1973, 90) construction
  line L574 (165.1973, 90) -> (155.1973, 90) construction
  line L575 (155.1973, 90) -> (155.1973, 86.825) construction
  line L576 (145.1973, 86.825) -> (155.1973, 86.825) construction
  line L577 (145.1973, 86.825) -> (145.1973, 90) construction
  line L578 (145.1973, 90) -> (135.1973, 90) construction
  line L579 (135.1973, 90) -> (135.1973, 86.825) construction
  line L580 (125.1973, 86.825) -> (135.1973, 86.825) construction
  line L581 (125.1973, 86.825) -> (125.1973, 90) construction
  line L582 (125.1973, 90) -> (115.1973, 90) construction
  line L583 (115.1973, 90) -> (115.1973, 86.825) construction
  line L584 (105.1973, 86.825) -> (115.1973, 86.825) construction
  line L585 (105.1973, 86.825) -> (105.1973, 90) construction
  line L586 (105.1973, 90) -> (95.1973, 90) construction
  line L587 (95.1973, 90) -> (95.1973, 86.825) construction
  line L588 (85.1973, 86.825) -> (95.1973, 86.825) construction
  line L589 (85.1973, 86.825) -> (85.1973, 90) construction
  line L590 (85.1973, 90) -> (75.1973, 90) construction
  line L591 (75.1973, 90) -> (75.1973, 86.825) construction
  line L592 (70.1973, 86.825) -> (75.1973, 86.825) construction
  line L593 (70.1973, 75) -> (70.1973, 86.825) construction
  line L594 (73.3723, 75) -> (70.1973, 75) construction
  line L595 (73.3723, 65) -> (73.3723, 75) construction
  line L596 (70.1973, 65) -> (73.3723, 65) construction
  line L597 (70.1973, 55) -> (70.1973, 65) construction
  line L598 (73.3723, 55) -> (70.1973, 55) construction
  line L599 (73.3723, 51.5) -> (73.3723, 55) construction
  line L600 (73.3723, 51.5) -> (75.3723, 51.5) construction
  line L601 (75.3723, 51.5) -> (75.3723, 52.75) construction
  line L602 (75.3723, 52.75) -> (77.8723, 52.75) construction
  line L603 (77.8723, 52.75) -> (77.8723, 51.5) construction
  line L604 (77.8723, 51.5) -> (84.1973, 51.5) construction
  line L605 (84.1973, 51.5) -> (84.1973, 48.5) construction
  line L606 (84.1973, 48.5) -> (77.8723, 48.5) construction
  line L607 (77.8723, 48.5) -> (77.8723, 47.25) construction
  line L608 (77.8723, 47.25) -> (75.3723, 47.25) construction
  line L609 (75.3723, 47.25) -> (75.3723, 48.5) construction
  line L610 (75.3723, 48.5) -> (73.3723, 48.5) construction
  line L611 (73.3723, 45) -> (73.3723, 48.5) construction
  line L612 (70.1973, 45) -> (73.3723, 45) construction
  line L613 (70.1973, 35) -> (70.1973, 45) construction
  line L614 (73.3723, 35) -> (70.1973, 35) construction
  line L615 (73.3723, 25) -> (73.3723, 35) construction
  line L616 (70.1973, 25) -> (73.3723, 25) construction
  line L617 (70.1973, 15) -> (70.1973, 25) construction
  line L618 (73.3723, 15) -> (70.1973, 15) construction
  line L619 (73.3723, 5) -> (73.3723, 15) construction
  line L620 (70.1973, 5) -> (73.3723, 5) construction
  line L621 (70.1973, -5) -> (70.1973, 5) construction
  line L622 (73.3723, -5) -> (70.1973, -5) construction
  line L623 (73.3723, -15) -> (73.3723, -5) construction
  line L624 (70.1973, -15) -> (73.3723, -15) construction
  line L625 (70.1973, -25) -> (70.1973, -15) construction
  line L626 (73.3723, -25) -> (70.1973, -25) construction
  line L627 (73.3723, -35) -> (73.3723, -25) construction
  line L628 (70.1973, -35) -> (73.3723, -35) construction
  line L629 (70.1973, -45) -> (70.1973, -35) construction
  line L630 (73.3723, -45) -> (70.1973, -45) construction
  line L631 (73.3723, -48.5) -> (73.3723, -45) construction
  line L632 (-316.5937, 75.1) -> (-316.5937, 86.925)
  line L633 (-316.5937, 86.925) -> (-314.7687, 86.925)
  line L634 (-314.7687, 86.925) -> (-314.7687, 90.1)
  line L635 (-314.7687, 90.1) -> (-304.5687, 90.1)
  line L636 (-304.5687, 90.1) -> (-304.5687, 86.925)
  line L637 (-304.5687, 86.925) -> (-294.7687, 86.925)
  line L638 (-294.7687, 86.925) -> (-294.7687, 90.1)
  line L639 (-294.7687, 90.1) -> (-284.5687, 90.1)
  line L640 (-284.5687, 90.1) -> (-284.5687, 86.925)
  line L641 (-284.5687, 86.925) -> (-274.7687, 86.925)
  line L642 (-274.7687, 86.925) -> (-274.7687, 90.1)
  line L643 (-274.7687, 90.1) -> (-264.5687, 90.1)
  line L644 (-264.5687, 90.1) -> (-264.5687, 86.925)
  line L645 (-264.5687, 86.925) -> (-254.7687, 86.925)
  line L646 (-254.7687, 86.925) -> (-254.7687, 90.1)
  line L647 (-254.7687, 90.1) -> (-244.5687, 90.1)
  line L648 (-244.5687, 90.1) -> (-244.5687, 86.925)
  line L649 (-244.5687, 86.925) -> (-234.7687, 86.925)
  line L650 (-234.7687, 86.925) -> (-234.7687, 90.1)
  line L651 (-234.7687, 90.1) -> (-224.5687, 90.1)
  line L652 (-224.5687, 90.1) -> (-224.5687, 86.925)
  line L653 (-224.5687, 86.925) -> (-214.7687, 86.925)
  line L654 (-214.7687, 86.925) -> (-214.7687, 90.1)
  line L655 (-214.7687, 90.1) -> (-204.5687, 90.1)
  line L656 (-204.5687, 90.1) -> (-204.5687, 86.925)
  line L657 (-204.5687, 86.925) -> (-202.7437, 86.925)
  line L658 (-202.7437, 86.925) -> (-202.7437, 75.1)
  line L659 (-202.7437, 75.1) -> (-199.5687, 75.1)
  line L660 (-199.5687, 75.1) -> (-199.5687, 64.9)
  line L661 (-199.5687, 64.9) -> (-202.7437, 64.9)
  line L662 (-202.7437, 64.9) -> (-202.7437, 55.1)
  line L663 (-202.7437, 55.1) -> (-199.5687, 55.1)
  line L664 (-199.5687, 55.1) -> (-199.5687, 44.9)
  line L665 (-199.5687, 44.9) -> (-202.7437, 44.9)
  line L666 (-202.7437, 44.9) -> (-202.7437, 35.1)
  line L667 (-202.7437, 35.1) -> (-199.5687, 35.1)
  line L668 (-199.5687, 35.1) -> (-199.5687, 24.9)
  line L669 (-199.5687, 24.9) -> (-202.7437, 24.9)
  line L670 (-202.7437, 24.9) -> (-202.7437, 15.1)
  line L671 (-202.7437, 15.1) -> (-199.5687, 15.1)
  line L672 (-199.5687, 15.1) -> (-199.5687, 4.9)
  line L673 (-199.5687, 4.9) -> (-202.7437, 4.9)
  line L674 (-202.7437, 4.9) -> (-202.7437, -4.9)
  line L675 (-202.7437, -4.9) -> (-199.5687, -4.9)
  line L676 (-199.5687, -4.9) -> (-199.5687, -15.1)
  line L677 (-199.5687, -15.1) -> (-202.7437, -15.1)
  line L678 (-202.7437, -15.1) -> (-202.7437, -24.9)
  line L679 (-202.7437, -24.9) -> (-199.5687, -24.9)
  line L680 (-199.5687, -24.9) -> (-199.5687, -35.1)
  line L681 (-199.5687, -35.1) -> (-202.7437, -35.1)
  line L682 (-202.7437, -35.1) -> (-202.7437, -44.9)
  line L683 (-202.7437, -44.9) -> (-199.5687, -44.9)
  line L684 (-199.5687, -44.9) -> (-199.5687, -55.1)
  line L685 (-199.5687, -55.1) -> (-202.7437, -55.1)
  line L686 (-202.7437, -55.1) -> (-202.7437, -64.9)
  line L687 (-202.7437, -64.9) -> (-199.5687, -64.9)
  line L688 (-199.5687, -64.9) -> (-199.5687, -75.1)
  line L689 (-199.5687, -75.1) -> (-202.7437, -75.1)
  line L690 (-202.7437, -75.1) -> (-202.7437, -86.925)
  line L691 (-202.7437, -86.925) -> (-204.5687, -86.925)
  line L692 (-204.5687, -86.925) -> (-204.5687, -90.1)
  line L693 (-204.5687, -90.1) -> (-214.7687, -90.1)
  line L694 (-214.7687, -90.1) -> (-214.7687, -86.925)
  line L695 (-214.7687, -86.925) -> (-224.5687, -86.925)
  line L696 (-224.5687, -86.925) -> (-224.5687, -90.1)
  line L697 (-224.5687, -90.1) -> (-234.7687, -90.1)
  line L698 (-234.7687, -90.1) -> (-234.7687, -86.925)
  line L699 (-234.7687, -86.925) -> (-244.5687, -86.925)
  line L700 (-244.5687, -86.925) -> (-244.5687, -90.1)
  line L701 (-244.5687, -90.1) -> (-254.7687, -90.1)
  line L702 (-254.7687, -90.1) -> (-254.7687, -86.925)
  line L703 (-254.7687, -86.925) -> (-264.5687, -86.925)
  line L704 (-264.5687, -86.925) -> (-264.5687, -90.1)
  line L705 (-264.5687, -90.1) -> (-274.7687, -90.1)
  line L706 (-274.7687, -90.1) -> (-274.7687, -86.925)
  line L707 (-274.7687, -86.925) -> (-284.5687, -86.925)
  line L708 (-284.5687, -86.925) -> (-284.5687, -90.1)
  line L709 (-284.5687, -90.1) -> (-294.7687, -90.1)
  line L710 (-294.7687, -90.1) -> (-294.7687, -86.925)
  line L711 (-294.7687, -86.925) -> (-304.5687, -86.925)
  line L712 (-304.5687, -86.925) -> (-304.5687, -90.1)
  line L713 (-304.5687, -90.1) -> (-314.7687, -90.1)
  line L714 (-314.7687, -90.1) -> (-314.7687, -86.925)
  line L715 (-314.7687, -86.925) -> (-316.5937, -86.925)
  line L716 (-316.5937, -86.925) -> (-316.5937, -75.1)
  line L717 (-316.5937, -75.1) -> (-319.7687, -75.1)
  line L718 (-319.7687, -75.1) -> (-319.7687, -64.9)
  line L719 (-319.7687, -64.9) -> (-316.5937, -64.9)
  line L720 (-316.5937, -64.9) -> (-316.5937, -55.1)
  line L721 (-316.5937, -55.1) -> (-319.7687, -55.1)
  line L722 (-319.7687, -55.1) -> (-319.7687, -44.9)
  line L723 (-319.7687, -44.9) -> (-316.5937, -44.9)
  line L724 (-316.5937, -44.9) -> (-316.5937, -35.1)
  line L725 (-316.5937, -35.1) -> (-319.7687, -35.1)
  line L726 (-319.7687, -35.1) -> (-319.7687, -24.9)
  line L727 (-319.7687, -24.9) -> (-316.5937, -24.9)
  line L728 (-316.5937, -24.9) -> (-316.5937, -15.1)
  line L729 (-316.5937, -15.1) -> (-319.7687, -15.1)
  line L730 (-319.7687, -15.1) -> (-319.7687, -4.9)
  line L731 (-319.7687, -4.9) -> (-316.5937, -4.9)
  line L732 (-316.5937, -4.9) -> (-316.5937, 4.9)
  line L733 (-316.5937, 4.9) -> (-319.7687, 4.9)
  line L734 (-319.7687, 4.9) -> (-319.7687, 15.1)
  line L735 (-319.7687, 15.1) -> (-316.5937, 15.1)
  line L736 (-316.5937, 15.1) -> (-316.5937, 24.9)
  line L737 (-316.5937, 24.9) -> (-319.7687, 24.9)
  line L738 (-319.7687, 24.9) -> (-319.7687, 35.1)
  line L739 (-319.7687, 35.1) -> (-316.5937, 35.1)
  line L740 (-316.5937, 35.1) -> (-316.5937, 44.9)
  line L741 (-316.5937, 44.9) -> (-319.7687, 44.9)
  line L742 (-319.7687, 44.9) -> (-319.7687, 55.1)
  line L743 (-319.7687, 55.1) -> (-316.5937, 55.1)
  line L744 (-316.5937, 55.1) -> (-316.5937, 64.9)
  line L745 (-316.5937, 64.9) -> (-319.7687, 64.9)
  line L746 (-319.7687, 64.9) -> (-319.7687, 75.1)
  line L747 (-319.7687, 75.1) -> (-316.5937, 75.1)
  line L748 (-304.7687, -14.9) -> (-304.7687, 14.9)
  line L749 (-304.7687, 14.9) -> (-314.5687, 14.9)
  line L750 (-314.5687, 14.9) -> (-314.5687, -14.9)
  line L751 (-314.5687, -14.9) -> (-304.7687, -14.9)
  line L752 (-214.5687, 14.9) -> (-214.5687, -14.9)
  line L753 (-214.5687, -14.9) -> (-204.7687, -14.9)
  line L754 (-204.7687, -14.9) -> (-204.7687, 14.9)
  line L755 (-204.7687, 14.9) -> (-214.5687, 14.9)
  line L756 (-175.8406, 86.925) -> (-166.0406, 86.925)
  line L757 (-166.0406, 86.925) -> (-166.0406, 90.1)
  line L758 (-166.0406, 90.1) -> (-155.8406, 90.1)
  line L759 (-155.8406, 90.1) -> (-155.8406, 86.925)
  line L760 (-155.8406, 86.925) -> (-146.0406, 86.925)
  line L761 (-146.0406, 86.925) -> (-146.0406, 90.1)
  line L762 (-146.0406, 90.1) -> (-135.8406, 90.1)
  line L763 (-135.8406, 90.1) -> (-135.8406, 86.925)
  line L764 (-135.8406, 86.925) -> (-126.0406, 86.925)
  line L765 (-126.0406, 86.925) -> (-126.0406, 90.1)
  line L766 (-126.0406, 90.1) -> (-115.8406, 90.1)
  line L767 (-115.8406, 90.1) -> (-115.8406, 86.925)
  line L768 (-115.8406, 86.925) -> (-106.0406, 86.925)
  line L769 (-106.0406, 86.925) -> (-106.0406, 90.1)
  line L770 (-106.0406, 90.1) -> (-95.8406, 90.1)
  line L771 (-95.8406, 90.1) -> (-95.8406, 86.925)
  line L772 (-95.8406, 86.925) -> (-86.0406, 86.925)
  line L773 (-86.0406, 86.925) -> (-86.0406, 90.1)
  line L774 (-86.0406, 90.1) -> (-75.8406, 90.1)
  line L775 (-75.8406, 90.1) -> (-75.8406, 86.925)
  line L776 (-75.8406, 86.925) -> (-70.8406, 86.925)
  line L777 (-70.8406, 86.925) -> (-70.8406, 74.9)
  line L778 (-70.8406, 74.9) -> (-74.0156, 74.9)
  line L779 (-74.0156, 74.9) -> (-74.0156, 65.1)
  line L780 (-74.0156, 65.1) -> (-70.8406, 65.1)
  line L781 (-70.8406, 65.1) -> (-70.8406, 54.9)
  line L782 (-70.8406, 54.9) -> (-74.0156, 54.9)
  line L783 (-74.0156, 54.9) -> (-74.0156, 51.4)
  line L784 (-74.0156, 51.4) -> (-76.2156, 51.4)
  line L785 (-76.2156, 51.4) -> (-76.2156, 52.65)
  line L786 (-76.2156, 52.65) -> (-78.5156, 52.65)
  line L787 (-78.5156, 52.65) -> (-78.5156, 51.4)
  line L788 (-78.5156, 51.4) -> (-84.8406, 51.4)
  line L789 (-84.8406, 51.4) -> (-84.8406, 48.6)
  line L790 (-84.8406, 48.6) -> (-78.5156, 48.6)
  line L791 (-78.5156, 48.6) -> (-78.5156, 47.35)
  line L792 (-78.5156, 47.35) -> (-76.2156, 47.35)
  line L793 (-76.2156, 47.35) -> (-76.2156, 48.6)
  line L794 (-76.2156, 48.6) -> (-74.0156, 48.6)
  line L795 (-74.0156, 48.6) -> (-74.0156, 45.1)
  line L796 (-74.0156, 45.1) -> (-70.8406, 45.1)
  line L797 (-70.8406, 45.1) -> (-70.8406, 34.9)
  line L798 (-70.8406, 34.9) -> (-74.0156, 34.9)
  line L799 (-74.0156, 34.9) -> (-74.0156, 25.1)
  line L800 (-74.0156, 25.1) -> (-70.8406, 25.1)
  line L801 (-70.8406, 25.1) -> (-70.8406, 14.9)
  line L802 (-70.8406, 14.9) -> (-74.0156, 14.9)
  line L803 (-74.0156, 14.9) -> (-74.0156, 5.1)
  line L804 (-74.0156, 5.1) -> (-70.8406, 5.1)
  line L805 (-70.8406, 5.1) -> (-70.8406, -5.1)
  line L806 (-70.8406, -5.1) -> (-74.0156, -5.1)
  line L807 (-74.0156, -5.1) -> (-74.0156, -14.9)
  line L808 (-74.0156, -14.9) -> (-70.8406, -14.9)
  line L809 (-70.8406, -14.9) -> (-70.8406, -25.1)
  line L810 (-70.8406, -25.1) -> (-74.0156, -25.1)
  line L811 (-74.0156, -25.1) -> (-74.0156, -34.9)
  line L812 (-74.0156, -34.9) -> (-70.8406, -34.9)
  line L813 (-70.8406, -34.9) -> (-70.8406, -45.1)
  line L814 (-70.8406, -45.1) -> (-74.0156, -45.1)
  line L815 (-74.0156, -45.1) -> (-74.0156, -48.6)
  line L816 (-74.0156, -48.6) -> (-76.2156, -48.6)
  line L817 (-76.2156, -48.6) -> (-76.2156, -47.35)
  line L818 (-76.2156, -47.35) -> (-78.5156, -47.35)
  line L819 (-78.5156, -47.35) -> (-78.5156, -48.6)
  line L820 (-78.5156, -48.6) -> (-84.8406, -48.6)
  line L821 (-84.8406, -48.6) -> (-84.8406, -51.4)
  line L822 (-84.8406, -51.4) -> (-78.5156, -51.4)
  line L823 (-78.5156, -51.4) -> (-78.5156, -52.65)
  line L824 (-78.5156, -52.65) -> (-76.2156, -52.65)
  line L825 (-76.2156, -52.65) -> (-76.2156, -51.4)
  line L826 (-76.2156, -51.4) -> (-74.0156, -51.4)
  line L827 (-74.0156, -51.4) -> (-74.0156, -54.9)
  line L828 (-74.0156, -54.9) -> (-70.8406, -54.9)
  line L829 (-70.8406, -54.9) -> (-70.8406, -65.1)
  line L830 (-70.8406, -65.1) -> (-74.0156, -65.1)
  line L831 (-74.0156, -65.1) -> (-74.0156, -74.9)
  line L832 (-74.0156, -74.9) -> (-70.8406, -74.9)
  line L833 (-70.8406, -74.9) -> (-70.8406, -86.925)
  line L834 (-70.8406, -86.925) -> (-75.8406, -86.925)
  line L835 (-75.8406, -86.925) -> (-75.8406, -90.1)
  line L836 (-75.8406, -90.1) -> (-86.0406, -90.1)